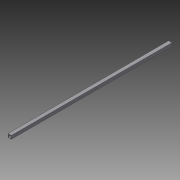
# Autodesk Inventor part: Push Rod
Saved by Autodesk Inventor 2014 SP1 (Build 180222100, 222)
## iProperties
Created: 2014-01-26
Part Number: Push Rod
Material: Generic
Document SubType Name: Modeling
Designer: tom
Density: 1 g/cm^3
Appearance: Default
Author: tom
Autodesk Inventor part; units mm, degrees
ref_plane "YZ Plane" through (0, 0, 0) normal (1, 0, 0) x (0, 1, 0)
ref_plane "XZ Plane" through (0, 0, 0) normal (0, 1, 0) x (-1, 0, 0)
ref_plane "XY Plane" through (0, 0, 0) normal (0, 0, 1) x (1, 0, 0)
sketch "Sketch1" plane through (0, 0, 0) normal (0, 0, 1) x (1, 0, 0)
  line L0 (-1.5875, 1.5875) -> (1.6078, 1.5875)
  line L1 (1.6078, 1.5875) -> (1.6078, -1.5875)
  line L2 (1.6078, -1.5875) -> (-1.5875, -1.5875)
  line L3 (-1.5875, -1.5875) -> (-1.5875, 1.5875)
  line L4 (1.2268, 1.2065) -> (-1.2065, 1.2065)
  line L5 (-1.2065, 1.2065) -> (-1.2065, -1.2065)
  line L6 (-1.2065, -1.2065) -> (1.2268, -1.2065)
  line L7 (1.2268, -1.2065) -> (1.2268, 1.2065)
  point P0 (0, 0)
  dimension "d0" = 1.5875
  dimension "d1" = 1.5875
  dimension "d2" = 3.1953
  dimension "d3" = 3.175
  dimension "d4" = 0.381
  dimension "d5" = 0.381
  dimension "d6" = 0.381
  dimension "d7" = 0.381
  constraints: 16 end point, 2 parallel, 1 horizontal, 1 perpendicular
  measures "d0" distance from line of point (0, 0) L3
  measures "d1" distance from line of point (0, 0) L0
  measures "d2" distance of L1.end L2.end
  measures "d3" distance of L0.end L1.end
  measures "d4" distance between parallel lines of L0 L4
  measures "d5" distance between parallel lines of L1 L7
  measures "d6" distance between parallel lines of L2 L6
  measures "d7" distance between parallel lines of L3 L5
extrude "Extrusion1" add sketch "Sketch1" along normal blind 152.4
body "Solid1"
